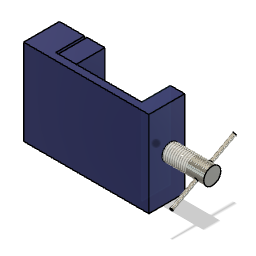
Vice v3 (Autodesk Fusion 360 design; units mm, degrees)
Autodesk Fusion 360 part; units mm, degrees
sketch "Sketch1" plane through (0, 0, 0) normal (0, 1, 0) x (1, 0, 0) in component "ViceBody"
  line L0 (87.5, -25) -> (-87.5, -25)
  line L1 (-87.5, -25) -> (-87.5, 25)
  line L2 (87.5, 25) -> (87.5, -25)
  line L3 (67.5, 25) -> (67.5, -15)
  line L4 (67.5, -15) -> (-52.5, -15)
  line L5 (-52.5, -15) -> (-52.5, 25)
  line L6 (-87.5, 25) -> (-52.5, 25)
  line L7 (67.5, 25) -> (87.5, 25)
  dimension "d1" = 175
  dimension "d2" = 50
  dimension "d3" = 40
  dimension "d4" = 35
  dimension "d5" = 20
  dimension "d6" = 25
  dimension "d7" = 87.5
  constraint horizontal L0
  constraint perpendicular L0 L1
  constraint parallel L0 L6
  constraint parallel L1 L2
  constraint vertical L3
  constraint horizontal L4
  constraint vertical L5
  constraint collinear L6 L7
  measures "d1" distance of L1.end L2.start
  measures "d2" distance of L0.end L1.end
  measures "d3" distance of L5.end L4.end
  measures "d4" distance of L1.end L5.end
  measures "d5" distance of L2.start L3.start
  measures "d6" distance of origin L0
  measures "d7" distance of origin L2
extrude "Extrude1" add sketch "Sketch1" along normal blind 120 makes body 1
sketch "Sketch1 (2)" plane through (0, 0, 15) normal (0, 0, -1) x (-1, 0, 0) in component "ViceSlide"
  line L0 (-67.5, 0) -> (52.5, 0)
  line L1 (52.5, 0) -> (52.5, 120)
  line L2 (52.5, 120) -> (-67.5, 120)
  line L3 (-67.5, 120) -> (-67.5, 0)
  line L4 (52.5, 120) -> (27.5, 120)
  line L5 (27.5, 120) -> (27.5, 0)
  line L6 (27.5, 0) -> (52.5, 0)
  line L7 (52.5, 0) -> (52.5, 120)
  point P0 (52.5, 120)
  dimension "d10" = 25
  constraint horizontal L4
  constraint vertical L5
  constraint horizontal L6
  constraint vertical L7
  constraint coincident L0 L5.end
  constraint coincident P0 L1.end
  measures "d10" distance of P0 L4.end
extrude "Extrude1'" add sketch "Sketch1 (2)" along normal blind 40 separate body contours L0 L1 L2 L4 L5 L6 L7 makes body 2 in component "ViceSlide"
sketch "Sketch1 (3)" plane through (67.5, 0, 0) normal (-1, 0, 0) x (0, 0, 1)
  line L0 (-25, 0) -> (15, 0)
  line L1 (15, 0) -> (15, 120)
  line L2 (15, 120) -> (-25, 120)
  line L3 (-25, 120) -> (-25, 0)
  point P0 (-5, 60)
  dimension "d13" = 20
  dimension "d14" = 60
  measures "d13" distance of L3 P0
  measures "d14" distance of L0 P0
hole "Hole1" at (67.5, 60, -5) direction (1, 0, 0) diameter 23.022 end up to surface (20 mm away) bodies 1
thread "Thread1" "ISO Metric profile 25.0 M25x2 6H"
sketch "Sketch2" plane through (-27.5, 0, 0) normal (1, 0, 0) x (0, 0, -1) in component "ViceSlide"
  line L0 (-15, 120) -> (-15, 0)
  line L1 (-15, 0) -> (25, 0)
  line L2 (25, 0) -> (25, 120)
  line L3 (25, 120) -> (-15, 120)
  circle A0 centre (5, 60) radius 11.5112
extrude "Extrude2" cut sketch "Sketch2" against normal blind 10 contours A0 bodies 2 in component "ViceSlide"
sketch "Sketch1 (4)" plane through (-27.5, 0, 0) normal (1, 0, 0) x (0, 0, -1) in component "Rod"
  circle A0 centre (5, 60) radius 11.5112
  line L0 (-15, 120) -> (-15, 0)
  line L1 (-15, 0) -> (25, 0)
  line L2 (25, 0) -> (25, 120)
  line L3 (25, 120) -> (-15, 120)
  circle A1 centre (5, 60) radius 11.5112
extrude "Extrude1''" add sketch "Sketch1 (4)" along normal blind 180 separate body contours A0 A1 makes body 3 in component "Rod"
thread "Thread1'" "ISO Metric profile 24.0 M24x3 4g6g" major diameter 23.7545 minor diameter 20.367 pitch 3 angle 60 resizes the face on face at (92.5, 59.4262, -16.4969) from (-22.5, 60, -5) to (127.5, 60, -5) on bodies 3 in component "Rod"
ref_plane "WorkPlane1" through (140.4841, 48.1227, -5) normal (0, -1, 0) x (0, 0, 1) in component "Rod"
sketch "Sketch2 (2)" plane through (140.4841, 48.1227, -5) normal (0, -1, 0) x (1, 0, 0) in component "Rod"
  circle A0 centre (0, 0) radius 2.5
  dimension "d25" = 5
  constraint coincident A0.centre origin
  measures "d25" diameter of A0
extrude "Extrude2'" cut sketch "Sketch2 (2)" against normal blind 24 bodies 3 in component "Rod"
sketch "Sketch1 (5)" plane through (0, 0, 0) normal (0, 1, 0) x (1, 0, 0) in component "Pin"
  circle A0 centre (0, 0) radius 2.5
  dimension "d28" = 5
  constraint coincident A0.centre origin
  measures "d28" diameter of A0
extrude "Extrude1'''" add sketch "Sketch1 (5)" along normal blind 100 separate body makes body 4 in component "Pin"
copy_body "CutPasteBodies1" bodies 1 removing the originals makes body 5 in component "ViceBody"
component "ViceBody" placed x (1, 0, 0) y (0, 1, 0) z (0, 0, 1) at (0, 0, 0)
component "ViceSlide" placed x (1, 0, 0) y (0, 1, 0) z (0, 0, 1) at (0.2151, 0, 0)
component "Rod" placed x (1, 0, 0) y (0, 1, 0) z (0, 0, 1) at (-9.7849, 0, 0)
component "Pin" placed x (1, 0, 0) y (0, 1, 0) z (0, 0, 1) at (130.6992, 11.121, -5)
